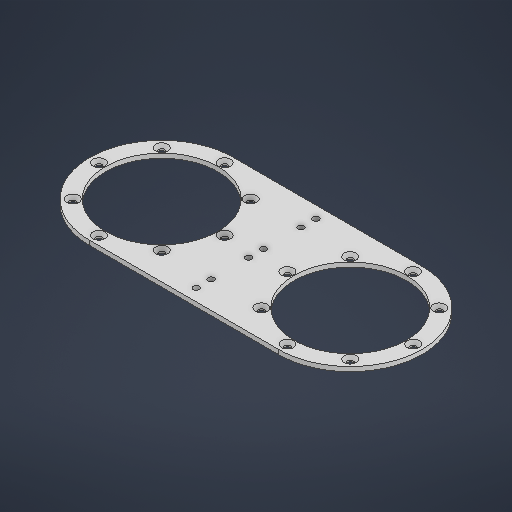
# Autodesk Inventor part: leg_connector
Saved by Autodesk Inventor 2026 (Build 300175000, 175)
## iProperties
Created: 2025-07-15
Part Number: leg_connector
Material: Generic
Document SubType Name: Modeling
Designer: User
Density: 1 g/cm^3
Appearance: Default
Author: User
Autodesk Inventor part; units mm, degrees
ref_plane "YZ Plane" through (0, 0, 0) normal (1, 0, 0) x (0, 1, 0)
ref_plane "XZ Plane" through (0, 0, 0) normal (0, 1, 0) x (-1, 0, 0)
ref_plane "XY Plane" through (0, 0, 0) normal (0, 0, 1) x (1, 0, 0)
sketch "Sketch1" plane through (0, 0, 0) normal (0, 1, 0) x (-1, 0, 0)
  arc A0 (-63, 48) -> (-63, -48) centre (-63, 0) ccw
  line L0 (0, -30.052) -> (0, -21.9885) construction
  circle A1 centre (-63, 0) radius 37.5
  circle A2 centre (-63, 0) radius 42 construction
  line L1 (-63, -48) -> (0, -48)
  line L2 (-63, 48) -> (0, 48)
  line L3 (0, 0) -> (-63, 0) construction
  circle A3 centre (-63, -42) radius 2
  circle A4 centre (-33.3015, -29.6985) radius 2
  circle A5 centre (-21, 0) radius 2
  circle A6 centre (-33.3015, 29.6985) radius 2
  circle A7 centre (-63, 42) radius 2
  circle A8 centre (-92.6985, 29.6985) radius 2
  circle A9 centre (-105, 0) radius 2
  circle A10 centre (-92.6985, -29.6985) radius 2
  arc A11 (63, -48) -> (63, 48) centre (63, 0) ccw
  circle A12 centre (63, 0) radius 37.5
  circle A13 centre (63, 0) radius 42 construction
  line L4 (63, -48) -> (0, -48)
  line L5 (63, 48) -> (0, 48)
  line L6 (0, 0) -> (63, 0) construction
  circle A14 centre (63, -42) radius 2
  circle A15 centre (33.3015, -29.6985) radius 2
  circle A16 centre (21, 0) radius 2
  circle A17 centre (33.3015, 29.6985) radius 2
  circle A18 centre (63, 42) radius 2
  circle A19 centre (92.6985, 29.6985) radius 2
  circle A20 centre (105, 0) radius 2
  circle A21 centre (92.6985, -29.6985) radius 2
  line L7 (0, 0) -> (0, -5) construction
  circle A22 centre (0, -5) radius 2
  line L8 (0, 0) -> (0, 5)
  circle A23 centre (0, 5) radius 2
  line L9 (0, -48) -> (0, -40) construction
  circle A24 centre (0, -40) radius 2
  line L10 (0, -40) -> (0, -30) construction
  circle A25 centre (0, -30) radius 2
  line L11 (0, 30.052) -> (0, 21.9885) construction
  line L12 (0, 48) -> (0, 40) construction
  circle A26 centre (0, 40) radius 2
  line L13 (0, 40) -> (0, 30) construction
  circle A27 centre (0, 30) radius 2
  dimension "d4" = 84
  dimension "d2" = 96
  dimension "d3" = 75
  dimension "d5" = 63
  dimension "d6" = 4
  dimension "d9" = 360
  dimension "d24" = 5
  dimension "d25" = 4
  dimension "d26" = 5
  dimension "d27" = 4
  dimension "d32" = 8
  dimension "d33" = 4
  dimension "d34" = 10
  dimension "d35" = 4
  constraints: 28 end point, 26 centre point, 19 symmetric about line, 10 coincident, 4 point on circle, 4 vertical, 3 horizontal, 2 point on line, 2 vertical alignment, 1 perpendicular, 1 tangent, 33 other
  measures "d2" diameter of A0
  measures "d3" diameter of A1
  measures "d5" distance of L3.start L3.end
  measures "d6" diameter of A3
  measures "d24" distance of L3.start L7.end
  measures "d25" diameter of A22
  measures "d26" distance of L3.start L8.end
  measures "d27" diameter of A23
  measures "d32" distance of L1.end L9.end
  measures "d33" diameter of A24
  measures "d34" distance of L10.start L10.end
  measures "d35" diameter of A25
extrude "Extrusion1" add sketch "Sketch1" along normal blind 3
chamfer "Chamfer1" distance 2 angle 45 16 edges at (-19, 3, 0) (-31.3015, 3, -29.6985) (-61, 3, -42) (-90.6985, 3, -29.6985) (-103, 3, 0) (-90.6985, 3, 29.6985) (-61, 3, 42) (-31.3015, 3, 29.6985) (35.3015, 3, 29.6985) (23, 3, 0) (35.3015, 3, -29.6985) (65, 3, -42) (94.6985, 3, -29.6985) (107, 3, 0) (94.6985, 3, 29.6985) (65, 3, 42)
body "Solid1"
